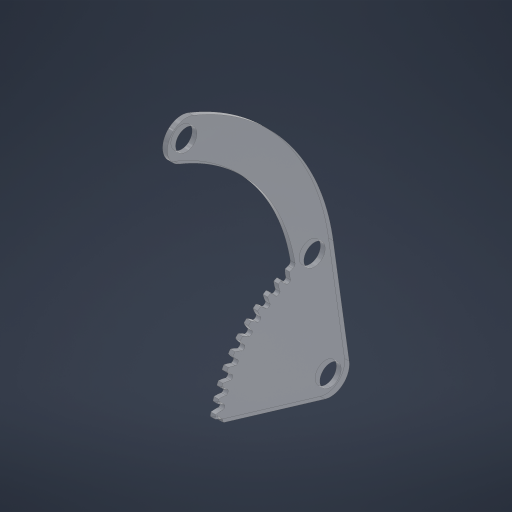
# Autodesk Inventor part: CORL_002_FanPlate
Saved by Autodesk Inventor 2024.2 (Build 282272000, 272)
## iProperties
Created: 2024-08-01
Part Number: CORL_002_FanPlate
Material: Polycarbonate, Clear
Document SubType Name: Modeling
Designer: Bryan
Mass: 349.383 g
Surface Area: 1019.32 cm^2
Volume: 291.153 cm^3
Density: 1.2 g/cm^3
Appearance: Polycarbonate - Clear
Author: Bryan
Autodesk Inventor part; units mm, degrees
ref_plane "YZ Plane" through (0, 0, 0) normal (1, 0, 0) x (0, 1, 0)
ref_plane "XZ Plane" through (0, 0, 0) normal (0, 1, 0) x (-1, 0, 0)
ref_plane "XY Plane" through (0, 0, 0) normal (0, 0, 1) x (1, 0, 0)
sketch "Sketch1" plane through (0, 0, 0) normal (1, 0, 0) x (0, 1, 0)
  circle A0 centre (0, 0) radius 152.4 construction
  circle A1 centre (0, 0) radius 157.48
  circle A2 centre (0, 0) radius 146.05
  line L0 (0, 0) -> (152.4, 0) construction
  line L1 (152.4, 0) -> (142.846, 36.9425) construction
  line L2 (142.846, 36.9425) -> (0, 0) construction
  arc A3 (147.5434, -0.8181) -> (142.846, 36.9425) centre (0, 0) ccw construction
  arc A4 (142.846, 36.9425) -> (137.6916, 53.0166) centre (0, 0) ccw construction
  line L3 (0, 0) -> (146, -3.8231) construction
  line L4 (137.6916, 53.0166) -> (157.4714, 1.6456) construction
  spline S0 degree 2 poles (157.4714, 1.6456) (152.4895, -0.3652) (147.5434, -0.8181) knots 0 0 0 1 1 1
  spline S1 degree 2 poles (157.1695, -9.8848) (152.2996, -7.616) (147.384, -6.9048) knots 0 0 0 1 1 1
  spline S2 degree 2 poles (156.4367, 18.0968) (151.6923, 15.5763) (146.8207, 14.6089) knots 0 0 0 1 1 1
  spline S3 degree 2 poles (157.3417, 6.5981) (152.2614, 8.3454) (147.2984, 8.5388) knots 0 0 0 1 1 1
  spline S4 degree 2 poles (153.6881, 34.3498) (149.2332, 31.3471) (144.4893, 29.8758) knots 0 0 0 1 1 1
  spline S5 degree 2 poles (155.7901, 23.0086) (150.555, 24.2153) (145.5989, 23.8889) knots 0 0 0 1 1 1
  spline S6 degree 2 poles (149.2557, 50.2264) (145.139, 46.7745) (140.575, 44.8154) knots 0 0 0 1 1 1
  spline S7 degree 2 poles (152.5316, 39.1671) (147.199, 39.8199) (142.3043, 38.9773) knots 0 0 0 1 1 1
  spline S8 degree 2 poles (143.188, 65.5527) (139.4546, 61.6895) (135.1204, 59.2639) knots 0 0 0 1 1 1
  spline S9 degree 2 poles (147.6019, 54.8964) (142.2303, 54.9883) (137.4505, 53.6386) knots 0 0 0 1 1 1
  spline S10 degree 2 poles (135.5514, 80.1608) (132.2424, 75.9285) (128.1854, 73.0632) knots 0 0 0 1 1 1
  spline S11 degree 2 poles (141.0551, 70.0243) (135.7033, 69.5542) (131.0907, 67.7123) knots 0 0 0 1 1 1
  spline S12 degree 2 poles (126.4298, 93.8907) (123.5812, 89.3356) (119.846, 86.062) knots 0 0 0 1 1 1
  spline S13 degree 2 poles (132.9629, 84.385) (127.6896, 83.358) (123.2948, 81.044) knots 0 0 0 1 1 1
  spline S14 degree 2 poles (115.9229, 106.5918) (113.5661, 101.764) (110.1936, 98.1178) knots 0 0 0 1 1 1
  spline S15 degree 2 poles (123.4139, 97.8211) (118.2768, 96.2485) (114.1479, 93.4879) knots 0 0 0 1 1 1
  spline S16 degree 2 poles (104.146, 118.1252) (102.3068, 113.0774) (99.3338, 109.0987) knots 0 0 0 1 1 1
  spline S17 degree 2 poles (112.5127, 110.1855) (107.5681, 108.0846) (103.7505, 104.9075) knots 0 0 0 1 1 1
  spline S18 degree 2 poles (91.2281, 128.3643) (89.9265, 123.1519) (87.3857, 118.8843) knots 0 0 0 1 1 1
  spline S19 degree 2 poles (100.3788, 121.3427) (95.6809, 118.7364) (92.2163, 115.1776) knots 0 0 0 1 1 1
  spline S20 degree 2 poles (77.3106, 137.197) (76.561, 131.8772) (74.4802, 127.3673) knots 0 0 0 1 1 1
  spline S21 degree 2 poles (87.1452, 131.1704) (82.7455, 128.0873) (79.6718, 124.1859) knots 0 0 0 1 1 1
  spline S22 degree 2 poles (62.5461, 144.5266) (62.3567, 139.1576) (60.7587, 134.4549) knots 0 0 0 1 1 1
  spline S23 degree 2 poles (72.9568, 139.561) (68.9034, 136.0349) (66.2544, 131.8336) knots 0 0 0 1 1 1
  spline S24 degree 2 poles (47.0963, 150.2727) (47.4691, 144.9133) (46.3715, 140.0693) knots 0 0 0 1 1 1
  spline S25 degree 2 poles (57.969, 146.4225) (54.3064, 142.4921) (52.1111, 138.0368) knots 0 0 0 1 1 1
  spline S26 degree 2 poles (31.1305, 154.3724) (32.0615, 149.0813) (31.4762, 144.1492) knots 0 0 0 1 1 1
  spline S27 degree 2 poles (42.3461, 151.6798) (39.1144, 147.3881) (37.3968, 142.7278) knots 0 0 0 1 1 1
  spline S28 degree 2 poles (14.8237, 156.7808) (16.3027, 151.616) (16.2361, 146.6497) knots 0 0 0 1 1 1
  spline S29 degree 2 poles (26.2593, 155.2752) (23.4939, 150.6692) (22.2728, 145.8549) knots 0 0 0 1 1 1
  spline S30 degree 2 poles (-1.6456, 157.4714) (0.3652, 152.4895) (0.8181, 147.5434) knots 0 0 0 1 1 1
  spline S31 degree 2 poles (9.8848, 157.1695) (7.616, 152.2996) (6.9048, 147.384) knots 0 0 0 1 1 1
  spline S32 degree 2 poles (-18.0968, 156.4367) (-15.5763, 151.6923) (-14.6089, 146.8207) knots 0 0 0 1 1 1
  spline S33 degree 2 poles (-6.5981, 157.3417) (-8.3454, 152.2614) (-8.5388, 147.2984) knots 0 0 0 1 1 1
  spline S34 degree 2 poles (-34.3498, 153.6881) (-31.3471, 149.2332) (-29.8758, 144.4893) knots 0 0 0 1 1 1
  spline S35 degree 2 poles (-23.0086, 155.7901) (-24.2153, 150.555) (-23.8889, 145.5989) knots 0 0 0 1 1 1
  spline S36 degree 2 poles (-50.2264, 149.2557) (-46.7745, 145.139) (-44.8154, 140.575) knots 0 0 0 1 1 1
  spline S37 degree 2 poles (-39.1671, 152.5316) (-39.8199, 147.199) (-38.9773, 142.3043) knots 0 0 0 1 1 1
  spline S38 degree 2 poles (-65.5527, 143.188) (-61.6895, 139.4546) (-59.2639, 135.1204) knots 0 0 0 1 1 1
  spline S39 degree 2 poles (-54.8964, 147.6019) (-54.9883, 142.2303) (-53.6386, 137.4505) knots 0 0 0 1 1 1
  spline S40 degree 2 poles (-80.1608, 135.5514) (-75.9285, 132.2424) (-73.0632, 128.1854) knots 0 0 0 1 1 1
  spline S41 degree 2 poles (-70.0243, 141.0551) (-69.5542, 135.7033) (-67.7123, 131.0907) knots 0 0 0 1 1 1
  spline S42 degree 2 poles (-93.8907, 126.4298) (-89.3356, 123.5812) (-86.062, 119.846) knots 0 0 0 1 1 1
  spline S43 degree 2 poles (-84.385, 132.9629) (-83.358, 127.6896) (-81.044, 123.2948) knots 0 0 0 1 1 1
  spline S44 degree 2 poles (-106.5918, 115.9229) (-101.764, 113.5661) (-98.1178, 110.1936) knots 0 0 0 1 1 1
  spline S45 degree 2 poles (-97.8211, 123.4139) (-96.2485, 118.2768) (-93.4879, 114.1479) knots 0 0 0 1 1 1
  spline S46 degree 2 poles (-118.1252, 104.146) (-113.0774, 102.3068) (-109.0987, 99.3338) knots 0 0 0 1 1 1
  spline S47 degree 2 poles (-110.1855, 112.5127) (-108.0846, 107.5681) (-104.9075, 103.7505) knots 0 0 0 1 1 1
  spline S48 degree 2 poles (-128.3643, 91.2281) (-123.1519, 89.9265) (-118.8843, 87.3857) knots 0 0 0 1 1 1
  spline S49 degree 2 poles (-121.3427, 100.3788) (-118.7364, 95.6809) (-115.1776, 92.2163) knots 0 0 0 1 1 1
  spline S50 degree 2 poles (-137.197, 77.3106) (-131.8772, 76.561) (-127.3673, 74.4802) knots 0 0 0 1 1 1
  spline S51 degree 2 poles (-131.1704, 87.1452) (-128.0873, 82.7455) (-124.1859, 79.6718) knots 0 0 0 1 1 1
  spline S52 degree 2 poles (-144.5266, 62.5461) (-139.1576, 62.3567) (-134.4549, 60.7587) knots 0 0 0 1 1 1
  spline S53 degree 2 poles (-139.561, 72.9568) (-136.0349, 68.9034) (-131.8336, 66.2544) knots 0 0 0 1 1 1
  spline S54 degree 2 poles (-150.2727, 47.0963) (-144.9133, 47.4691) (-140.0693, 46.3715) knots 0 0 0 1 1 1
  spline S55 degree 2 poles (-146.4225, 57.969) (-142.4921, 54.3064) (-138.0368, 52.1111) knots 0 0 0 1 1 1
  spline S56 degree 2 poles (-154.3724, 31.1305) (-149.0813, 32.0615) (-144.1492, 31.4762) knots 0 0 0 1 1 1
  spline S57 degree 2 poles (-151.6798, 42.3461) (-147.3881, 39.1144) (-142.7278, 37.3968) knots 0 0 0 1 1 1
  spline S58 degree 2 poles (-156.7808, 14.8237) (-151.616, 16.3027) (-146.6497, 16.2361) knots 0 0 0 1 1 1
  spline S59 degree 2 poles (-155.2752, 26.2593) (-150.6692, 23.4939) (-145.8549, 22.2728) knots 0 0 0 1 1 1
  spline S60 degree 2 poles (-157.4714, -1.6456) (-152.4895, 0.3652) (-147.5434, 0.8181) knots 0 0 0 1 1 1
  spline S61 degree 2 poles (-157.1695, 9.8848) (-152.2996, 7.616) (-147.384, 6.9048) knots 0 0 0 1 1 1
  spline S62 degree 2 poles (-156.4367, -18.0968) (-151.6923, -15.5763) (-146.8207, -14.6089) knots 0 0 0 1 1 1
  spline S63 degree 2 poles (-157.3417, -6.5981) (-152.2614, -8.3454) (-147.2984, -8.5388) knots 0 0 0 1 1 1
  spline S64 degree 2 poles (-153.6881, -34.3498) (-149.2332, -31.3471) (-144.4893, -29.8758) knots 0 0 0 1 1 1
  spline S65 degree 2 poles (-155.7901, -23.0086) (-150.555, -24.2153) (-145.5989, -23.8889) knots 0 0 0 1 1 1
  spline S66 degree 2 poles (-149.2557, -50.2264) (-145.139, -46.7745) (-140.575, -44.8154) knots 0 0 0 1 1 1
  spline S67 degree 2 poles (-152.5316, -39.1671) (-147.199, -39.8199) (-142.3043, -38.9773) knots 0 0 0 1 1 1
  spline S68 degree 2 poles (-143.188, -65.5527) (-139.4546, -61.6895) (-135.1204, -59.2639) knots 0 0 0 1 1 1
  spline S69 degree 2 poles (-147.6019, -54.8964) (-142.2303, -54.9883) (-137.4505, -53.6386) knots 0 0 0 1 1 1
  spline S70 degree 2 poles (-135.5514, -80.1608) (-132.2424, -75.9285) (-128.1854, -73.0632) knots 0 0 0 1 1 1
  spline S71 degree 2 poles (-141.0551, -70.0243) (-135.7033, -69.5542) (-131.0907, -67.7123) knots 0 0 0 1 1 1
  spline S72 degree 2 poles (-126.4298, -93.8907) (-123.5812, -89.3356) (-119.846, -86.062) knots 0 0 0 1 1 1
  spline S73 degree 2 poles (-132.9629, -84.385) (-127.6896, -83.358) (-123.2948, -81.044) knots 0 0 0 1 1 1
  spline S74 degree 2 poles (-115.9229, -106.5918) (-113.5661, -101.764) (-110.1936, -98.1178) knots 0 0 0 1 1 1
  spline S75 degree 2 poles (-123.4139, -97.8211) (-118.2768, -96.2485) (-114.1479, -93.4879) knots 0 0 0 1 1 1
  spline S76 degree 2 poles (-104.146, -118.1252) (-102.3068, -113.0774) (-99.3338, -109.0987) knots 0 0 0 1 1 1
  spline S77 degree 2 poles (-112.5127, -110.1855) (-107.5681, -108.0846) (-103.7505, -104.9075) knots 0 0 0 1 1 1
  spline S78 degree 2 poles (-91.2281, -128.3643) (-89.9265, -123.1519) (-87.3857, -118.8843) knots 0 0 0 1 1 1
  spline S79 degree 2 poles (-100.3788, -121.3427) (-95.6809, -118.7364) (-92.2163, -115.1776) knots 0 0 0 1 1 1
  spline S80 degree 2 poles (-77.3106, -137.197) (-76.561, -131.8772) (-74.4802, -127.3673) knots 0 0 0 1 1 1
  spline S81 degree 2 poles (-87.1452, -131.1704) (-82.7455, -128.0873) (-79.6718, -124.1859) knots 0 0 0 1 1 1
  spline S82 degree 2 poles (-62.5461, -144.5266) (-62.3567, -139.1576) (-60.7587, -134.4549) knots 0 0 0 1 1 1
  spline S83 degree 2 poles (-72.9568, -139.561) (-68.9034, -136.0349) (-66.2544, -131.8336) knots 0 0 0 1 1 1
  spline S84 degree 2 poles (-47.0963, -150.2727) (-47.4691, -144.9133) (-46.3715, -140.0693) knots 0 0 0 1 1 1
  spline S85 degree 2 poles (-57.969, -146.4225) (-54.3064, -142.4921) (-52.1111, -138.0368) knots 0 0 0 1 1 1
  spline S86 degree 2 poles (-31.1305, -154.3724) (-32.0615, -149.0813) (-31.4762, -144.1492) knots 0 0 0 1 1 1
  spline S87 degree 2 poles (-42.3461, -151.6798) (-39.1144, -147.3881) (-37.3968, -142.7278) knots 0 0 0 1 1 1
  spline S88 degree 2 poles (-14.8237, -156.7808) (-16.3027, -151.616) (-16.2361, -146.6497) knots 0 0 0 1 1 1
  spline S89 degree 2 poles (-26.2593, -155.2752) (-23.4939, -150.6692) (-22.2728, -145.8549) knots 0 0 0 1 1 1
  spline S90 degree 2 poles (1.6456, -157.4714) (-0.3652, -152.4895) (-0.8181, -147.5434) knots 0 0 0 1 1 1
  spline S91 degree 2 poles (-9.8848, -157.1695) (-7.616, -152.2996) (-6.9048, -147.384) knots 0 0 0 1 1 1
  spline S92 degree 2 poles (18.0968, -156.4367) (15.5763, -151.6923) (14.6089, -146.8207) knots 0 0 0 1 1 1
  spline S93 degree 2 poles (6.5981, -157.3417) (8.3454, -152.2614) (8.5388, -147.2984) knots 0 0 0 1 1 1
  spline S94 degree 2 poles (34.3498, -153.6881) (31.3471, -149.2332) (29.8758, -144.4893) knots 0 0 0 1 1 1
  spline S95 degree 2 poles (23.0086, -155.7901) (24.2153, -150.555) (23.8889, -145.5989) knots 0 0 0 1 1 1
  spline S96 degree 2 poles (50.2264, -149.2557) (46.7745, -145.139) (44.8154, -140.575) knots 0 0 0 1 1 1
  spline S97 degree 2 poles (39.1671, -152.5316) (39.8199, -147.199) (38.9773, -142.3043) knots 0 0 0 1 1 1
  spline S98 degree 2 poles (65.5527, -143.188) (61.6895, -139.4546) (59.2639, -135.1204) knots 0 0 0 1 1 1
  spline S99 degree 2 poles (54.8964, -147.6019) (54.9883, -142.2303) (53.6386, -137.4505) knots 0 0 0 1 1 1
  spline S100 degree 2 poles (80.1608, -135.5514) (75.9285, -132.2424) (73.0632, -128.1854) knots 0 0 0 1 1 1
  spline S101 degree 2 poles (70.0243, -141.0551) (69.5542, -135.7033) (67.7123, -131.0907) knots 0 0 0 1 1 1
  spline S102 degree 2 poles (93.8907, -126.4298) (89.3356, -123.5812) (86.062, -119.846) knots 0 0 0 1 1 1
  spline S103 degree 2 poles (84.385, -132.9629) (83.358, -127.6896) (81.044, -123.2948) knots 0 0 0 1 1 1
  spline S104 degree 2 poles (106.5918, -115.9229) (101.764, -113.5661) (98.1178, -110.1936) knots 0 0 0 1 1 1
  spline S105 degree 2 poles (97.8211, -123.4139) (96.2485, -118.2768) (93.4879, -114.1479) knots 0 0 0 1 1 1
  spline S106 degree 2 poles (118.1252, -104.146) (113.0774, -102.3068) (109.0987, -99.3338) knots 0 0 0 1 1 1
  spline S107 degree 2 poles (110.1855, -112.5127) (108.0846, -107.5681) (104.9075, -103.7505) knots 0 0 0 1 1 1
  spline S108 degree 2 poles (128.3643, -91.2281) (123.1519, -89.9265) (118.8843, -87.3857) knots 0 0 0 1 1 1
  spline S109 degree 2 poles (121.3427, -100.3788) (118.7364, -95.6809) (115.1776, -92.2163) knots 0 0 0 1 1 1
  spline S110 degree 2 poles (137.197, -77.3106) (131.8772, -76.561) (127.3673, -74.4802) knots 0 0 0 1 1 1
  spline S111 degree 2 poles (131.1704, -87.1452) (128.0873, -82.7455) (124.1859, -79.6718) knots 0 0 0 1 1 1
  spline S112 degree 2 poles (144.5266, -62.5461) (139.1576, -62.3567) (134.4549, -60.7587) knots 0 0 0 1 1 1
  spline S113 degree 2 poles (139.561, -72.9568) (136.0349, -68.9034) (131.8336, -66.2544) knots 0 0 0 1 1 1
  spline S114 degree 2 poles (150.2727, -47.0963) (144.9133, -47.4691) (140.0693, -46.3715) knots 0 0 0 1 1 1
  spline S115 degree 2 poles (146.4225, -57.969) (142.4921, -54.3064) (138.0368, -52.1111) knots 0 0 0 1 1 1
  spline S116 degree 2 poles (154.3724, -31.1305) (149.0813, -32.0615) (144.1492, -31.4762) knots 0 0 0 1 1 1
  spline S117 degree 2 poles (151.6798, -42.3461) (147.3881, -39.1144) (142.7278, -37.3968) knots 0 0 0 1 1 1
  spline S118 degree 2 poles (156.7808, -14.8237) (151.616, -16.3027) (146.6497, -16.2361) knots 0 0 0 1 1 1
  spline S119 degree 2 poles (155.2752, -26.2593) (150.6692, -23.4939) (145.8549, -22.2728) knots 0 0 0 1 1 1
  arc A5 (147.5434, -0.8181) -> (147.384, -6.9048) centre (149.8956, -3.9252) ccw
  arc A6 (146.8207, 14.6089) -> (147.2984, 8.5388) centre (149.4847, 11.7647) ccw
  arc A7 (144.4893, 29.8758) -> (145.5989, 23.8889) centre (147.4361, 27.3257) ccw
  arc A8 (140.575, 44.8154) -> (142.3043, 38.9773) centre (143.7721, 42.5872) ccw
  arc A9 (135.1204, 59.2639) -> (137.4505, 53.6386) centre (138.5329, 57.3822) ccw
  arc A10 (128.1854, 73.0632) -> (131.0907, 67.7123) centre (131.776, 71.5485) ccw
  arc A11 (119.846, 86.062) -> (123.2948, 81.044) centre (123.5752, 84.9309) ccw
  arc A12 (110.1936, 98.1178) -> (114.1479, 93.4879) centre (114.0206, 97.3828) ccw
  arc A13 (99.3338, 109.0987) -> (103.7505, 104.9075) centre (103.2167, 108.7677) ccw
  arc A14 (87.3857, 118.8843) -> (92.2163, 115.1776) centre (91.2819, 118.9609) ccw
  arc A15 (74.4802, 127.3673) -> (79.6718, 124.1859) centre (78.3471, 127.8508) ccw
  arc A16 (60.7587, 134.4549) -> (66.2544, 131.8336) centre (64.5538, 135.3399) ccw
  arc A17 (46.3715, 140.0693) -> (52.1111, 138.0368) centre (50.0533, 141.3462) ccw
  arc A18 (31.4762, 144.1492) -> (37.3968, 142.7278) centre (35.0044, 145.8039) ccw
  arc A19 (16.2361, 146.6497) -> (22.2728, 145.8549) centre (19.572, 148.6641) ccw
  arc A20 (0.8181, 147.5434) -> (6.9048, 147.384) centre (3.9252, 149.8956) ccw
  arc A21 (-14.6089, 146.8207) -> (-8.5388, 147.2984) centre (-11.7647, 149.4847) ccw
  arc A22 (-29.8758, 144.4893) -> (-23.8889, 145.5989) centre (-27.3257, 147.4361) ccw
  arc A23 (-44.8154, 140.575) -> (-38.9773, 142.3043) centre (-42.5872, 143.7721) ccw
  arc A24 (-59.2639, 135.1204) -> (-53.6386, 137.4505) centre (-57.3822, 138.5329) ccw
  arc A25 (-73.0632, 128.1854) -> (-67.7123, 131.0907) centre (-71.5485, 131.776) ccw
  arc A26 (-86.062, 119.846) -> (-81.044, 123.2948) centre (-84.9309, 123.5752) ccw
  arc A27 (-98.1178, 110.1936) -> (-93.4879, 114.1479) centre (-97.3828, 114.0206) ccw
  arc A28 (-109.0987, 99.3338) -> (-104.9075, 103.7505) centre (-108.7677, 103.2167) ccw
  arc A29 (-118.8843, 87.3857) -> (-115.1776, 92.2163) centre (-118.9609, 91.2819) ccw
  arc A30 (-127.3673, 74.4802) -> (-124.1859, 79.6718) centre (-127.8508, 78.3471) ccw
  arc A31 (-134.4549, 60.7587) -> (-131.8336, 66.2544) centre (-135.3399, 64.5538) ccw
  arc A32 (-140.0693, 46.3715) -> (-138.0368, 52.1111) centre (-141.3462, 50.0533) ccw
  arc A33 (-144.1492, 31.4762) -> (-142.7278, 37.3968) centre (-145.8039, 35.0044) ccw
  arc A34 (-146.6497, 16.2361) -> (-145.8549, 22.2728) centre (-148.6641, 19.572) ccw
  arc A35 (-147.5434, 0.8181) -> (-147.384, 6.9048) centre (-149.8956, 3.9252) ccw
  arc A36 (-146.8207, -14.6089) -> (-147.2984, -8.5388) centre (-149.4847, -11.7647) ccw
  arc A37 (-144.4893, -29.8758) -> (-145.5989, -23.8889) centre (-147.4361, -27.3257) ccw
  arc A38 (-140.575, -44.8154) -> (-142.3043, -38.9773) centre (-143.7721, -42.5872) ccw
  arc A39 (-135.1204, -59.2639) -> (-137.4505, -53.6386) centre (-138.5329, -57.3822) ccw
  arc A40 (-128.1854, -73.0632) -> (-131.0907, -67.7123) centre (-131.776, -71.5485) ccw
  arc A41 (-119.846, -86.062) -> (-123.2948, -81.044) centre (-123.5752, -84.9309) ccw
  arc A42 (-110.1936, -98.1178) -> (-114.1479, -93.4879) centre (-114.0206, -97.3828) ccw
  arc A43 (-99.3338, -109.0987) -> (-103.7505, -104.9075) centre (-103.2167, -108.7677) ccw
  arc A44 (-87.3857, -118.8843) -> (-92.2163, -115.1776) centre (-91.2819, -118.9609) ccw
  arc A45 (-74.4802, -127.3673) -> (-79.6718, -124.1859) centre (-78.3471, -127.8508) ccw
  arc A46 (-60.7587, -134.4549) -> (-66.2544, -131.8336) centre (-64.5538, -135.3399) ccw
  arc A47 (-46.3715, -140.0693) -> (-52.1111, -138.0368) centre (-50.0533, -141.3462) ccw
  arc A48 (-31.4762, -144.1492) -> (-37.3968, -142.7278) centre (-35.0044, -145.8039) ccw
  arc A49 (-16.2361, -146.6497) -> (-22.2728, -145.8549) centre (-19.572, -148.6641) ccw
  arc A50 (-0.8181, -147.5434) -> (-6.9048, -147.384) centre (-3.9252, -149.8956) ccw
  arc A51 (14.6089, -146.8207) -> (8.5388, -147.2984) centre (11.7647, -149.4847) ccw
  arc A52 (29.8758, -144.4893) -> (23.8889, -145.5989) centre (27.3257, -147.4361) ccw
  arc A53 (44.8154, -140.575) -> (38.9773, -142.3043) centre (42.5872, -143.7721) ccw
  arc A54 (59.2639, -135.1204) -> (53.6386, -137.4505) centre (57.3822, -138.5329) ccw
  arc A55 (73.0632, -128.1854) -> (67.7123, -131.0907) centre (71.5485, -131.776) ccw
  arc A56 (86.062, -119.846) -> (81.044, -123.2948) centre (84.9309, -123.5752) ccw
  arc A57 (98.1178, -110.1936) -> (93.4879, -114.1479) centre (97.3828, -114.0206) ccw
  arc A58 (109.0987, -99.3338) -> (104.9075, -103.7505) centre (108.7677, -103.2167) ccw
  arc A59 (118.8843, -87.3857) -> (115.1776, -92.2163) centre (118.9609, -91.2819) ccw
  arc A60 (127.3673, -74.4802) -> (124.1859, -79.6718) centre (127.8508, -78.3471) ccw
  arc A61 (134.4549, -60.7587) -> (131.8336, -66.2544) centre (135.3399, -64.5538) ccw
  arc A62 (140.0693, -46.3715) -> (138.0368, -52.1111) centre (141.3462, -50.0533) ccw
  arc A63 (144.1492, -31.4762) -> (142.7278, -37.3968) centre (145.8039, -35.0044) ccw
  arc A64 (146.6497, -16.2361) -> (145.8549, -22.2728) centre (148.6641, -19.572) ccw
  point P0 (152.1911, -7.976)
  point P1 (151.5651, 15.9301)
  point P2 (152.1911, 7.976)
  point P3 (149.0697, 31.6857)
  point P4 (150.5237, 23.8406)
  point P5 (144.941, 47.0942)
  point P6 (147.2071, 39.444)
  point P7 (139.2243, 61.9867)
  point P8 (142.2777, 54.6153)
  point P9 (131.9823, 76.2)
  point P10 (135.7894, 69.1882)
  point P11 (123.2942, 89.5785)
  point P12 (127.8134, 83.003)
  point P13 (113.2553, 101.9755)
  point P14 (118.437, 95.9084)
  point P15 (101.9755, 113.2553)
  point P16 (107.7631, 107.7631)
  point P17 (89.5785, 123.2942)
  point P18 (95.9084, 118.437)
  point P19 (76.2, 131.9823)
  point P20 (83.003, 127.8134)
  point P21 (61.9867, 139.2243)
  point P22 (69.1882, 135.7894)
  point P23 (47.0942, 144.941)
  point P24 (54.6153, 142.2777)
  point P25 (31.6857, 149.0697)
  point P26 (39.444, 147.2071)
  point P27 (15.9301, 151.5651)
  point P28 (23.8406, 150.5237)
  point P29 (0, 152.4)
  point P30 (7.976, 152.1911)
  point P31 (-15.9301, 151.5651)
  point P32 (-7.976, 152.1911)
  point P33 (-31.6857, 149.0697)
  point P34 (-23.8406, 150.5237)
  point P35 (-47.0942, 144.941)
  point P36 (-39.444, 147.2071)
  point P37 (-61.9867, 139.2243)
  point P38 (-54.6153, 142.2777)
  point P39 (-76.2, 131.9823)
  point P40 (-69.1882, 135.7894)
  point P41 (-89.5785, 123.2942)
  point P42 (-83.003, 127.8134)
  point P43 (-101.9755, 113.2553)
  point P44 (-95.9084, 118.437)
  point P45 (-113.2553, 101.9755)
  point P46 (-107.7631, 107.7631)
  point P47 (-123.2942, 89.5785)
  point P48 (-118.437, 95.9084)
  point P49 (-131.9823, 76.2)
  point P50 (-127.8134, 83.003)
  point P51 (-139.2243, 61.9867)
  point P52 (-135.7894, 69.1882)
  point P53 (-144.941, 47.0942)
  point P54 (-142.2777, 54.6153)
  point P55 (-149.0697, 31.6857)
  point P56 (-147.2071, 39.444)
  point P57 (-151.5651, 15.9301)
  point P58 (-150.5237, 23.8406)
  point P59 (-152.4, 0)
  point P60 (-152.1911, 7.976)
  point P61 (-151.5651, -15.9301)
  point P62 (-152.1911, -7.976)
  point P63 (-149.0697, -31.6857)
  point P64 (-150.5237, -23.8406)
  point P65 (-144.941, -47.0942)
  point P66 (-147.2071, -39.444)
  point P67 (-139.2243, -61.9867)
  point P68 (-142.2777, -54.6153)
  point P69 (-131.9823, -76.2)
  point P70 (-135.7894, -69.1882)
  point P71 (-123.2942, -89.5785)
  point P72 (-127.8134, -83.003)
  point P73 (-113.2553, -101.9755)
  point P74 (-118.437, -95.9084)
  point P75 (-101.9755, -113.2553)
  point P76 (-107.7631, -107.7631)
  point P77 (-89.5785, -123.2942)
  point P78 (-95.9084, -118.437)
  point P79 (-76.2, -131.9823)
  point P80 (-83.003, -127.8134)
  point P81 (-61.9867, -139.2243)
  point P82 (-69.1882, -135.7894)
  point P83 (-47.0942, -144.941)
  point P84 (-54.6153, -142.2777)
  point P85 (-31.6857, -149.0697)
  point P86 (-39.444, -147.2071)
  point P87 (-15.9301, -151.5651)
  point P88 (-23.8406, -150.5237)
  point P89 (0, -152.4)
  point P90 (-7.976, -152.1911)
  point P91 (15.9301, -151.5651)
  point P92 (7.976, -152.1911)
  point P93 (31.6857, -149.0697)
  point P94 (23.8406, -150.5237)
  point P95 (47.0942, -144.941)
  point P96 (39.444, -147.2071)
  point P97 (61.9867, -139.2243)
  point P98 (54.6153, -142.2777)
  point P99 (76.2, -131.9823)
  point P100 (69.1882, -135.7894)
  point P101 (89.5785, -123.2942)
  point P102 (83.003, -127.8134)
  point P103 (101.9755, -113.2553)
  point P104 (95.9084, -118.437)
  point P105 (113.2553, -101.9755)
  point P106 (107.7631, -107.7631)
  point P107 (123.2942, -89.5785)
  point P108 (118.437, -95.9084)
  point P109 (131.9823, -76.2)
  point P110 (127.8134, -83.003)
  point P111 (139.2243, -61.9867)
  point P112 (135.7894, -69.1882)
  point P113 (144.941, -47.0942)
  point P114 (142.2777, -54.6153)
  point P115 (149.0697, -31.6857)
  point P116 (147.2071, -39.444)
  point P117 (151.5651, -15.9301)
  point P118 (150.5237, -23.8406)
  point P119 (-110.1573, 193.0296)
  point P120 (-157.4714, -1.6456)
  point P121 (157.1695, -9.8848)
  point P122 (222.1508, -6.6412)
  point P123 (222.2472, -1.1158)
  point P124 (157.3417, 6.5981)
  point P125 (222.0729, 8.8715)
  point P126 (221.7837, 14.3901)
  point P127 (155.7901, 23.0086)
  point P128 (220.9131, 24.3409)
  point P129 (220.2396, 29.8259)
  point P130 (152.5316, 39.1671)
  point P131 (218.677, 39.6917)
  point P132 (217.6226, 45.1163)
  point P133 (149.2557, 50.2264)
  point P134 (147.6019, 54.8964)
  point P135 (215.3756, 54.8491)
  point P136 (213.9453, 60.187)
  point P137 (143.188, 65.5527)
  point P138 (141.0551, 70.0243)
  point P139 (211.0248, 69.7394)
  point P140 (209.2257, 74.9645)
  point P141 (135.5514, 80.1608)
  point P142 (132.9629, 84.385)
  point P143 (205.646, 84.2898)
  point P144 (203.4868, 89.3767)
  point P145 (126.4298, 93.8907)
  point P146 (123.4139, 97.8211)
  point P147 (199.2653, 98.4297)
  point P148 (196.7565, 103.3535)
  point P149 (115.9229, 106.5918)
  point P150 (112.5127, 110.1855)
  point P151 (191.9138, 112.0899)
  point P152 (189.0676, 116.8268)
  point P153 (104.146, 118.1252)
  point P154 (100.3788, 121.3427)
  point P155 (183.6273, 125.2041)
  point P156 (180.4576, 129.7309)
  point P157 (91.2281, 128.3643)
  point P158 (87.1452, 131.1704)
  point P159 (174.4462, 137.7083)
  point P160 (170.9685, 142.003)
  point P161 (77.3106, 137.197)
  point P162 (72.9568, 139.561)
  point P163 (164.4152, 149.5416)
  point P164 (160.6464, 153.5832)
  point P165 (62.5461, 144.5266)
  point P166 (57.969, 146.4225)
  point P167 (153.5832, 160.6464)
  point P168 (149.5416, 164.4152)
  point P169 (47.0963, 150.2727)
  point P170 (42.3461, 151.6798)
  point P171 (142.003, 170.9685)
  point P172 (137.7083, 174.4462)
  point P173 (31.1305, 154.3724)
  point P174 (26.2593, 155.2752)
  point P175 (129.7309, 180.4576)
  point P176 (125.2041, 183.6273)
  point P177 (14.8237, 156.7808)
  point P178 (9.8848, 157.1695)
  point P179 (116.8268, 189.0676)
  point P180 (112.0899, 191.9138)
  point P181 (-1.6456, 157.4714)
  point P182 (-6.5981, 157.3417)
  point P183 (103.3535, 196.7565)
  point P184 (98.4297, 199.2653)
  point P185 (-18.0968, 156.4367)
  point P186 (-23.0086, 155.7901)
  point P187 (89.3767, 203.4868)
  point P188 (84.2898, 205.646)
  point P189 (-34.3498, 153.6881)
  point P190 (-39.1671, 152.5316)
  point P191 (74.9645, 209.2257)
  point P192 (69.7394, 211.0248)
  point P193 (-54.8964, 147.6019)
  point P194 (60.187, 213.9453)
  point P195 (54.8491, 215.3756)
  point P196 (-65.5527, 143.188)
  point P197 (-70.0243, 141.0551)
  point P198 (45.1163, 217.6226)
  point P199 (39.6917, 218.677)
  dimension "d18" = 304.8
  dimension "d19" = 314.96
  dimension "d20" = 292.1
  dimension "d21" = 14.5
  dimension "d22" = 38.1579
  dimension "d23" = 38.1579
  dimension "d26" = 1.5
  dimension "d61" = 55.0474
  dimension "d62" = 16.8895
  dimension "d65" = 360
  dimension "d104" = 360
  constraints: 184 point on circle, 62 centre point, 10 end point, 3 coincident, 3 symmetric about line, 2 tangent, 1 horizontal, 1 horizontal alignment, 1 perpendicular, 1154 other
  measures "d21" angle of L0 L2
  measures "d22" distance of L0.end L1.end
  measures "d26" angle of L3 L0
  measures "d61" distance of L4.start L4.end
extrude "Extrusion2" add sketch "Sketch1" along normal blind 6.35 contours S0 A5 A2 A6 S3 A1 | A1 S118 A64 A2 A5 S1 | S2 A6 A2 A7 S5 A1 | A2 | A1 S116 A63 A2 A64 S119 | S4 A7 A2 A8 S7 A1 | A63 S117 A1 S114 A62 A2 | A2 A9 S9 A1 S6 A8 | A62 S115 A1 S112 A61 A2 | A2 A10 S11 A1 S8 A9 | A61 S113 A1 S110 A60 A2 | A2 A11 S13 A1 S10 A10 | A60 S111 A1 S108 A59 A2 | A60 S110 A1 S111 | A2 A12 S15 A1 S12 A11 | A59 S109 A1 S106 A58 A2 | A59 S108 A1 S109 | A2 A13 S17 A1 S14 A12 | A58 S107 A1 S104 A57 A2 | A58 S106 A1 S107 | A2 A14 S19 A1 S16 A13 | A57 S105 A1 S102 A56 A2 | A57 S104 A1 S105 | A2 A15 S21 A1 S18 A14 | A56 S103 A1 S100 A55 A2 | A56 S102 A1 S103 | A2 A16 S23 A1 S20 A15 | A55 S101 A1 S98 A54 A2 | A55 S100 A1 S101 | A2 A17 S25 A1 S22 A16 | A54 S99 A1 S96 A53 A2 | A54 S98 A1 S99 | A2 A18 S27 A1 S24 A17 | A53 S97 A1 S94 A52 A2 | A53 S96 A1 S97 | A2 A19 S29 A1 S26 A18 | A52 S95 A1 S92 A51 A2 | A52 S94 A1 S95 | A2 A20 S31 A1 S28 A19 | A51 S93 A1 S90 A50 A2 | A51 S92 A1 S93 | A2 A21 S33 A1 S30 A20 | A50 S91 A1 S88 A49 A2 | A50 S90 A1 S91 | A2 A22 S35 A1 S32 A21 | A49 S89 A1 S86 A48 A2 | A49 S88 A1 S89 | A2 A23 S37 A1 S34 A22 | A22 S34 A1 S35 | A48 S87 A1 S84 A47 A2 | A48 S86 A1 S87 | A2 A24 S39 A1 S36 A23 | A23 S36 A1 S37 | A47 S85 A1 S82 A46 A2 | A47 S84 A1 S85 | A2 A25 S41 A1 S38 A24 | A24 S38 A1 S39 | A46 S83 A1 S80 A45 A2 | A46 S82 A1 S83 | A2 A26 S43 A1 S40 A25 | A25 S40 A1 S41 | A45 S81 A1 S78 A44 A2 | A45 S80 A1 S81 | A2 A27 S45 A1 S42 A26 | A26 S42 A1 S43 | A44 S79 A1 S76 A43 A2 | A44 S78 A1 S79 | A2 A28 S47 A1 S44 A27 | A27 S44 A1 S45 | A43 S77 A1 S74 A42 A2 | A43 S76 A1 S77 | A2 A29 S49 A1 S46 A28 | A28 S46 A1 S47 | A42 S75 A1 S72 A41 A2 | A42 S74 A1 S75 | A2 A30 S51 A1 S48 A29 | A29 S48 A1 S49 | A41 S73 A1 S70 A40 A2 | A41 S72 A1 S73 | A2 A31 S53 A1 S50 A30 | A30 S50 A1 S51 | A40 S71 A1 S68 A39 A2 | A40 S70 A1 S71 | A2 A32 S55 A1 S52 A31 | A31 S52 A1 S53 | A39 S69 A1 S66 A38 A2 | A39 S68 A1 S69 | A2 A33 S57 A1 S54 A32 | A32 S54 A1 S55 | A38 S67 A1 S64 A37 A2 | A38 S66 A1 S67 | A2 A34 S59 A1 S56 A33 | A33 S56 A1 S57 | A37 S65 A1 S62 A36 A2 | A37 S64 A1 S65 | A2 A35 S61 A1 S58 A34 | A34 S58 A1 S59 | A36 S63 A1 S60 A35 A2 | A36 S62 A1 S63 | A35 S60 A1 S61
sketch "Sketch11" plane through (6.35, 0, 0) normal (1, 0, 0) x (0, 0, -1)
  arc A0 (-1.6456, 157.4714) -> (-6.5981, 157.3417) centre (0, 0) ccw projected
  arc A1 (0.8181, 147.5434) -> (6.9048, 147.384) centre (3.9252, 149.8956) ccw projected
  line L0 (3.8231, 146) -> (0, 0) construction
  line L1 (0, 0) -> (-156.4677, 17.8272) construction
  circle A2 centre (0, 0) radius 157.48
  arc A3 (-146.6497, 16.2361) -> (-145.8549, 22.2728) centre (-148.6641, 19.572) ccw projected
  arc A4 (-156.4367, -18.0968) -> (72.9568, 139.561) centre (0, 0) ccw projected
  arc A5 (60.7587, 134.4549) -> (66.2544, 131.8336) centre (64.5538, 135.3399) ccw projected
  arc A6 (62.5461, 144.5266) -> (57.969, 146.4225) centre (0, 0) ccw projected
  arc A7 (46.3715, 140.0693) -> (52.1111, 138.0368) centre (50.0533, 141.3462) ccw projected
  arc A8 (47.0963, 150.2727) -> (42.3461, 151.6798) centre (0, 0) ccw projected
  arc A9 (31.4762, 144.1492) -> (37.3968, 142.7278) centre (35.0044, 145.8039) ccw projected
  arc A10 (31.1305, 154.3724) -> (26.2593, 155.2752) centre (0, 0) ccw projected
  arc A11 (16.2361, 146.6497) -> (22.2728, 145.8549) centre (19.572, 148.6641) ccw projected
  arc A12 (14.8237, 156.7808) -> (9.8848, 157.1695) centre (0, 0) ccw projected
  arc A13 (0.8181, 147.5434) -> (6.9048, 147.384) centre (3.9252, 149.8956) ccw projected
  spline S0 degree 2 poles (0.8181, 147.5434) (0.3652, 152.4895) (-1.6456, 157.4714) knots 0 0 0 1 1 1 projected
  arc A14 (-1.6456, 157.4714) -> (-6.5981, 157.3417) centre (0, 0) ccw projected
  spline S1 degree 2 poles (-6.5981, 157.3417) (-8.3454, 152.2614) (-8.5388, 147.2984) knots 0 0 0 1 1 1 projected
  arc A15 (-14.6089, 146.8207) -> (-8.5388, 147.2984) centre (-11.7647, 149.4847) ccw projected
  spline S2 degree 2 poles (-14.6089, 146.8207) (-15.5763, 151.6923) (-18.0968, 156.4367) knots 0 0 0 1 1 1 projected
  arc A16 (-18.0968, 156.4367) -> (-23.0086, 155.7901) centre (0, 0) ccw projected
  spline S3 degree 2 poles (-23.0086, 155.7901) (-24.2153, 150.555) (-23.8889, 145.5989) knots 0 0 0 1 1 1 projected
  arc A17 (-29.8758, 144.4893) -> (-23.8889, 145.5989) centre (-27.3257, 147.4361) ccw projected
  spline S4 degree 2 poles (-29.8758, 144.4893) (-31.3471, 149.2332) (-34.3498, 153.6881) knots 0 0 0 1 1 1 projected
  arc A18 (-34.3498, 153.6881) -> (-39.1671, 152.5316) centre (0, 0) ccw projected
  spline S5 degree 2 poles (-39.1671, 152.5316) (-39.8199, 147.199) (-38.9773, 142.3043) knots 0 0 0 1 1 1 projected
  arc A19 (-44.8154, 140.575) -> (-38.9773, 142.3043) centre (-42.5872, 143.7721) ccw projected
  spline S6 degree 2 poles (-44.8154, 140.575) (-46.7745, 145.139) (-50.2264, 149.2557) knots 0 0 0 1 1 1 projected
  arc A20 (-50.2264, 149.2557) -> (-54.8964, 147.6019) centre (0, 0) ccw projected
  spline S7 degree 2 poles (-54.8964, 147.6019) (-54.9883, 142.2303) (-53.6386, 137.4505) knots 0 0 0 1 1 1 projected
  arc A21 (-59.2639, 135.1204) -> (-53.6386, 137.4505) centre (-57.3822, 138.5329) ccw projected
  spline S8 degree 2 poles (-59.2639, 135.1204) (-61.6895, 139.4546) (-65.5527, 143.188) knots 0 0 0 1 1 1 projected
  arc A22 (-65.5527, 143.188) -> (-70.0243, 141.0551) centre (0, 0) ccw projected
  spline S9 degree 2 poles (-70.0243, 141.0551) (-69.5542, 135.7033) (-67.7123, 131.0907) knots 0 0 0 1 1 1 projected
  arc A23 (-73.0632, 128.1854) -> (-67.7123, 131.0907) centre (-71.5485, 131.776) ccw projected
  spline S10 degree 2 poles (-73.0632, 128.1854) (-75.9285, 132.2424) (-80.1608, 135.5514) knots 0 0 0 1 1 1 projected
  arc A24 (-80.1608, 135.5514) -> (-84.385, 132.9629) centre (0, 0) ccw projected
  spline S11 degree 2 poles (-84.385, 132.9629) (-83.358, 127.6896) (-81.044, 123.2948) knots 0 0 0 1 1 1 projected
  arc A25 (-86.062, 119.846) -> (-81.044, 123.2948) centre (-84.9309, 123.5752) ccw projected
  spline S12 degree 2 poles (-86.062, 119.846) (-89.3356, 123.5812) (-93.8907, 126.4298) knots 0 0 0 1 1 1 projected
  arc A26 (-93.8907, 126.4298) -> (-97.8211, 123.4139) centre (0, 0) ccw projected
  spline S13 degree 2 poles (-97.8211, 123.4139) (-96.2485, 118.2768) (-93.4879, 114.1479) knots 0 0 0 1 1 1 projected
  arc A27 (-98.1178, 110.1936) -> (-93.4879, 114.1479) centre (-97.3828, 114.0206) ccw projected
  spline S14 degree 2 poles (-98.1178, 110.1936) (-101.764, 113.5661) (-106.5918, 115.9229) knots 0 0 0 1 1 1 projected
  arc A28 (-106.5918, 115.9229) -> (-110.1855, 112.5127) centre (0, 0) ccw projected
  spline S15 degree 2 poles (-110.1855, 112.5127) (-108.0846, 107.5681) (-104.9075, 103.7505) knots 0 0 0 1 1 1 projected
  arc A29 (-109.0987, 99.3338) -> (-104.9075, 103.7505) centre (-108.7677, 103.2167) ccw projected
  spline S16 degree 2 poles (-109.0987, 99.3338) (-113.0774, 102.3068) (-118.1252, 104.146) knots 0 0 0 1 1 1 projected
  arc A30 (-118.1252, 104.146) -> (-121.3427, 100.3788) centre (0, 0) ccw projected
  spline S17 degree 2 poles (-121.3427, 100.3788) (-118.7364, 95.6809) (-115.1776, 92.2163) knots 0 0 0 1 1 1 projected
  arc A31 (-118.8843, 87.3857) -> (-115.1776, 92.2163) centre (-118.9609, 91.2819) ccw projected
  spline S18 degree 2 poles (-118.8843, 87.3857) (-123.1519, 89.9265) (-128.3643, 91.2281) knots 0 0 0 1 1 1 projected
  arc A32 (-128.3643, 91.2281) -> (-131.1704, 87.1452) centre (0, 0) ccw projected
  spline S19 degree 2 poles (-131.1704, 87.1452) (-128.0873, 82.7455) (-124.1859, 79.6718) knots 0 0 0 1 1 1 projected
  arc A33 (-127.3673, 74.4802) -> (-124.1859, 79.6718) centre (-127.8508, 78.3471) ccw projected
  spline S20 degree 2 poles (-127.3673, 74.4802) (-131.8772, 76.561) (-137.197, 77.3106) knots 0 0 0 1 1 1 projected
  arc A34 (-137.197, 77.3106) -> (-139.561, 72.9568) centre (0, 0) ccw projected
  spline S21 degree 2 poles (-139.561, 72.9568) (-136.0349, 68.9034) (-131.8336, 66.2544) knots 0 0 0 1 1 1 projected
  arc A35 (-134.4549, 60.7587) -> (-131.8336, 66.2544) centre (-135.3399, 64.5538) ccw projected
  spline S22 degree 2 poles (-134.4549, 60.7587) (-139.1576, 62.3567) (-144.5266, 62.5461) knots 0 0 0 1 1 1 projected
  arc A36 (-144.5266, 62.5461) -> (-146.4225, 57.969) centre (0, 0) ccw projected
  spline S23 degree 2 poles (-146.4225, 57.969) (-142.4921, 54.3064) (-138.0368, 52.1111) knots 0 0 0 1 1 1 projected
  arc A37 (-140.0693, 46.3715) -> (-138.0368, 52.1111) centre (-141.3462, 50.0533) ccw projected
  spline S24 degree 2 poles (-140.0693, 46.3715) (-144.9133, 47.4691) (-150.2727, 47.0963) knots 0 0 0 1 1 1 projected
  arc A38 (-150.2727, 47.0963) -> (-151.6798, 42.3461) centre (0, 0) ccw projected
  spline S25 degree 2 poles (-151.6798, 42.3461) (-147.3881, 39.1144) (-142.7278, 37.3968) knots 0 0 0 1 1 1 projected
  arc A39 (-144.1492, 31.4762) -> (-142.7278, 37.3968) centre (-145.8039, 35.0044) ccw projected
  spline S26 degree 2 poles (-144.1492, 31.4762) (-149.0813, 32.0615) (-154.3724, 31.1305) knots 0 0 0 1 1 1 projected
  arc A40 (-154.3724, 31.1305) -> (-155.2752, 26.2593) centre (0, 0) ccw projected
  spline S27 degree 2 poles (-155.2752, 26.2593) (-150.6692, 23.4939) (-145.8549, 22.2728) knots 0 0 0 1 1 1 projected
  arc A41 (-146.6497, 16.2361) -> (-145.8549, 22.2728) centre (-148.6641, 19.572) ccw projected
  arc A42 (-156.7808, 14.8237) -> (-157.1695, 9.8848) centre (0, 0) ccw projected
  arc A43 (-147.5434, 0.8181) -> (-147.384, 6.9048) centre (-149.8956, 3.9252) ccw projected
  arc A44 (-157.4714, -1.6456) -> (-157.3417, -6.5981) centre (0, 0) ccw projected
  arc A45 (-146.8207, -14.6089) -> (-147.2984, -8.5388) centre (-149.4847, -11.7647) ccw projected
  arc A46 (-144.1492, 31.4762) -> (-142.7278, 37.3968) centre (-145.8039, 35.0044) ccw projected
  circle A47 centre (0, 0) radius 14.2875
  circle A48 centre (0, 0) radius 25.4
  line L2 (-143.0357, 16.3365) -> (-7.2895, -24.3315)
  line L3 (3.8231, 146) -> (25.12, 3.7611)
  line L4 (-144.8005, 19.0634) -> (-145.1333, 16.5358) construction
  arc A49 (-144.8005, 19.0634) -> (-142.6003, 16.2473) centre (-142.3168, 18.7364) ccw
  point P0 (57.969, 146.4225)
  point P1 (47.0963, 150.2727)
  point P2 (42.3461, 151.6798)
  point P3 (31.1305, 154.3724)
  point P4 (26.2593, 155.2752)
  point P5 (14.8237, 156.7808)
  point P6 (9.8848, 157.1695)
  point P7 (6.9048, 147.384)
  point P8 (-146.6497, 16.2361)
  point P9 (-156.7808, 14.8237)
  point P10 (-157.1695, 9.8848)
  point P11 (-157.4714, -1.6456)
  point P12 (-157.3417, -6.5981)
  point P13 (72.9568, 139.561)
  point P14 (-146.0914, 16.645)
  point P15 (-151.6798, 42.3461)
  point P16 (-146.4225, 57.969)
  point P17 (-139.561, 72.9568)
  point P18 (-131.1704, 87.1452)
  point P19 (-121.3427, 100.3788)
  point P20 (-110.1855, 112.5127)
  point P21 (-97.8211, 123.4139)
  point P22 (-84.385, 132.9629)
  point P23 (-70.0243, 141.0551)
  point P24 (-54.8964, 147.6019)
  point P25 (-39.1671, 152.5316)
  point P26 (-50.2264, 149.2557)
  point P27 (-23.0086, 155.7901)
  point P28 (-34.3498, 153.6881)
  point P29 (-1.6456, 157.4714)
  point P30 (-155.2752, 26.2593)
  point P31 (-6.5981, 157.3417)
  point P32 (-18.0968, 156.4367)
  point P33 (26.2593, 155.2752)
  point P34 (14.8237, 156.7808)
  point P35 (9.8848, 157.1695)
  point P36 (-156.7808, 14.8237)
  point P37 (-157.1695, 9.8848)
  point P38 (-157.4714, -1.6456)
  point P39 (-157.3417, -6.5981)
  point P40 (72.9568, 139.561)
  point P41 (57.969, 146.4225)
  point P42 (47.0963, 150.2727)
  point P43 (42.3461, 151.6798)
  point P44 (31.1305, 154.3724)
  point P45 (-153.6233, 31.255)
  point P46 (0.8181, 147.5434)
  point P47 (0.6649, 25.3913)
  point P48 (-25.2367, 2.8754)
  point P49 (-151.6798, 42.3461)
  point P50 (-155.2752, 26.2593)
  point P51 (-1.6456, 157.4714)
  point P52 (-6.5981, 157.3417)
  point P53 (-18.0968, 156.4367)
  point P54 (-23.0086, 155.7901)
  point P55 (-34.3498, 153.6881)
  point P56 (-39.1671, 152.5316)
  point P57 (-50.2264, 149.2557)
  point P58 (-54.8964, 147.6019)
  point P59 (-70.0243, 141.0551)
  point P60 (-84.385, 132.9629)
  point P61 (-97.8211, 123.4139)
  point P62 (-110.1855, 112.5127)
  point P63 (-121.3427, 100.3788)
  point P64 (-131.1704, 87.1452)
  point P65 (-139.561, 72.9568)
  point P66 (-146.4225, 57.969)
  point P67 (-145.8549, 22.2728)
  dimension "d106" = 314.96
  dimension "d107" = 85
  dimension "d108" = 28.575
  dimension "d109" = 50.8
  constraints: 10 end point, 9 point on circle, 6 tangent, 3 centre point, 3 coincident, 3 point on line, 44 other
  measures "d107" angle of L0 L1
  measures "d108" diameter of A47
  measures "d109" diameter of A48
extrude "Extrusion12" cut sketch "Sketch11" against normal blind 6.35 contours A2 S27 A3 A49 L2 A48 L3 A1 S0 | S1 A15 S2 A2 | S3 A17 S4 A2 | S5 A19 S6 A2 | S7 A21 S8 A2 | S9 A23 S10 A2 | A2 S25 A39 S26 | S11 A25 S12 A2 | A2 S23 A37 S24 | S13 A27 S14 A2 | A2 S21 A35 S22 | S15 A29 S16 A2 | A2 S19 A33 S20 | S17 A31 S18 A2 | A47
sketch "Sketch14" plane through (6.35, 0, 0) normal (1, 0, 0) x (0, 0, -1)
  arc A0 (0.8181, 147.5434) -> (3.8231, 146) centre (3.9252, 149.8956) ccw projected
  line L0 (0, 0) -> (3.8231, 146) construction
  line L1 (0, 0) -> (-47.8481, 150.035) construction
  arc A1 (-50.2264, 149.2557) -> (-54.8964, 147.6019) centre (0, 0) ccw projected
  circle A2 centre (-21.4577, 150.8818) radius 25.4
  circle A3 centre (-21.4577, 150.8818) radius 14.2875
  dimension "d110" = 19.188
  dimension "d111" = 50.8
  dimension "d112" = 28.575
  constraints: 4 end point, 2 centre point, 2 tangent, 1 coincident, 1 point on circle
  measures "d110" angle of L0 L1
  measures "d111" diameter of A2
  measures "d112" diameter of A3
extrude "Extrusion14" add sketch "Sketch14" against normal blind 6.35
extrude "Extrusion15" cut sketch "Sketch14" against normal blind 6.35 contours A3
sketch "Sketch17" plane through (6.35, 0, 0) normal (1, 0, 0) x (0, 0, -1)
  arc A0 (3.4736, 146.0249) -> (-44.6138, 140.4435) centre (-21.4577, 150.8818) ccw projected
  arc A1 (-50.2264, 149.2557) -> (-46.7086, 153.6299) centre (-51.8881, 154.1936) ccw
  arc A2 (-50.2264, 149.2557) -> (-54.8964, 147.6019) centre (0, 0) ccw projected
  circle A3 centre (-21.4577, 150.8818) radius 14.2875 projected
  circle A4 centre (0, 0) radius 14.2875 projected
  arc A5 (3.4736, 146.0249) -> (-44.6138, 140.4435) centre (-21.4577, 150.8818) ccw projected
  arc A6 (-44.8154, 140.575) -> (-44.6138, 140.4435) centre (-42.5872, 143.7721) ccw projected
  spline S0 degree 2 poles (-44.8154, 140.575) (-46.7745, 145.139) (-50.2264, 149.2557) knots 0 0 0 1 1 1 projected
  arc A7 (-50.2264, 149.2557) -> (-54.8964, 147.6019) centre (0, 0) ccw projected
  arc A8 (-59.2639, 135.1204) -> (-53.6386, 137.4505) centre (-57.3822, 138.5329) ccw projected
  arc A9 (-65.5527, 143.188) -> (-70.0243, 141.0551) centre (0, 0) ccw projected
  arc A10 (-73.0632, 128.1854) -> (-67.7123, 131.0907) centre (-71.5485, 131.776) ccw projected
  arc A11 (-80.1608, 135.5514) -> (-84.385, 132.9629) centre (0, 0) ccw projected
  arc A12 (-86.062, 119.846) -> (-81.044, 123.2948) centre (-84.9309, 123.5752) ccw projected
  arc A13 (-93.8907, 126.4298) -> (-97.8211, 123.4139) centre (0, 0) ccw projected
  arc A14 (-98.1178, 110.1936) -> (-93.4879, 114.1479) centre (-97.3828, 114.0206) ccw projected
  arc A15 (-106.5918, 115.9229) -> (-110.1855, 112.5127) centre (0, 0) ccw projected
  arc A16 (-109.0987, 99.3338) -> (-104.9075, 103.7505) centre (-108.7677, 103.2167) ccw projected
  arc A17 (-118.1252, 104.146) -> (-121.3427, 100.3788) centre (0, 0) ccw projected
  arc A18 (-118.8843, 87.3857) -> (-115.1776, 92.2163) centre (-118.9609, 91.2819) ccw projected
  arc A19 (-128.3643, 91.2281) -> (-131.1704, 87.1452) centre (0, 0) ccw projected
  arc A20 (-127.3673, 74.4802) -> (-124.1859, 79.6718) centre (-127.8508, 78.3471) ccw projected
  arc A21 (-137.197, 77.3106) -> (-139.561, 72.9568) centre (0, 0) ccw projected
  arc A22 (-134.4549, 60.7587) -> (-131.8336, 66.2544) centre (-135.3399, 64.5538) ccw projected
  arc A23 (-144.5266, 62.5461) -> (-146.4225, 57.969) centre (0, 0) ccw projected
  arc A24 (-140.0693, 46.3715) -> (-138.0368, 52.1111) centre (-141.3462, 50.0533) ccw projected
  arc A25 (-150.2727, 47.0963) -> (-151.6798, 42.3461) centre (0, 0) ccw projected
  arc A26 (-144.1492, 31.4762) -> (-142.7278, 37.3968) centre (-145.8039, 35.0044) ccw projected
  line L0 (-143.0357, 16.3365) -> (-7.2895, -24.3315) projected
  arc A27 (-7.2895, -24.3315) -> (25.12, 3.7611) centre (0, 0) ccw projected
  line L1 (25.12, 3.7611) -> (3.8231, 146) projected
  arc A28 (3.4736, 146.0249) -> (3.8231, 146) centre (3.9252, 149.8956) ccw projected
  line L2 (3.6892, 154.4581) -> (25.147, 3.5763)
  arc A29 (-7.2895, -24.3315) -> (25.12, 3.7611) centre (0, 0) ccw projected
  arc A30 (-154.3724, 31.1305) -> (-155.2752, 26.2593) centre (0, 0) ccw projected
  arc A31 (-144.8005, 19.0634) -> (-145.8549, 22.2728) centre (-148.6641, 19.572) ccw projected
  arc A32 (-144.8005, 19.0634) -> (-143.0357, 16.3365) centre (-142.3168, 18.7364) ccw projected
  point P0 (3.4736, 146.0249)
  point P1 (-50.2264, 149.2557)
  point P2 (-44.6138, 140.4435)
  constraints: 5 point on circle, 4 tangent, 2 end point, 1 centre point, 22 other
extrude "Extrusion18" add sketch "Sketch17" against normal blind 6.35 contours A0 L2 L1 A28 | A0 A6 S0 A1
sketch "Sketch20" plane through (6.35, 0, 0) normal (1, 0, 0) x (0, 0, -1)
  circle A0 centre (-21.4577, 150.8818) radius 14.2875 construction
  line L0 (-21.4577, 150.8818) -> (-193.8348, 370.7693) construction
  line L1 (-21.4577, 150.8818) -> (0, 0) construction
  circle A1 centre (-193.8348, 370.7693) radius 14.2875
  circle A2 centre (-193.8348, 370.7693) radius 25.4 construction
  arc A3 (-21.4577, 150.8818) -> (-193.8348, 370.7693) centre (-298.0744, 111.5427) ccw construction
  arc A4 (-46.6047, 147.3055) -> (-203.3111, 347.2033) centre (-298.0744, 111.5427) ccw
  arc A5 (3.6892, 154.4581) -> (-184.3585, 394.3354) centre (-298.0744, 111.5427) ccw
  line L2 (-46.6047, 147.3055) -> (3.6892, 154.4581)
  arc A6 (-184.3585, 394.3354) -> (-203.3111, 347.2033) centre (-193.8348, 370.7693) ccw
  circle A7 centre (-21.4577, 150.8818) radius 14.2875 projected
  circle A8 centre (0, 0) radius 14.2875 projected
  arc A9 (3.6892, 154.4581) -> (-46.7086, 153.6299) centre (-21.4577, 150.8818) ccw projected
  arc A10 (-50.2264, 149.2557) -> (-46.7086, 153.6299) centre (-51.8881, 154.1936) ccw projected
  arc A11 (-50.2264, 149.2557) -> (-54.8964, 147.6019) centre (0, 0) ccw projected
  arc A12 (-59.2639, 135.1204) -> (-53.6386, 137.4505) centre (-57.3822, 138.5329) ccw projected
  arc A13 (-65.5527, 143.188) -> (-70.0243, 141.0551) centre (0, 0) ccw projected
  arc A14 (-73.0632, 128.1854) -> (-67.7123, 131.0907) centre (-71.5485, 131.776) ccw projected
  arc A15 (-80.1608, 135.5514) -> (-84.385, 132.9629) centre (0, 0) ccw projected
  arc A16 (-86.062, 119.846) -> (-81.044, 123.2948) centre (-84.9309, 123.5752) ccw projected
  arc A17 (-93.8907, 126.4298) -> (-97.8211, 123.4139) centre (0, 0) ccw projected
  arc A18 (-98.1178, 110.1936) -> (-93.4879, 114.1479) centre (-97.3828, 114.0206) ccw projected
  arc A19 (-106.5918, 115.9229) -> (-110.1855, 112.5127) centre (0, 0) ccw projected
  arc A20 (-109.0987, 99.3338) -> (-104.9075, 103.7505) centre (-108.7677, 103.2167) ccw projected
  arc A21 (-118.1252, 104.146) -> (-121.3427, 100.3788) centre (0, 0) ccw projected
  arc A22 (-118.8843, 87.3857) -> (-115.1776, 92.2163) centre (-118.9609, 91.2819) ccw projected
  arc A23 (-128.3643, 91.2281) -> (-131.1704, 87.1452) centre (0, 0) ccw projected
  arc A24 (-127.3673, 74.4802) -> (-124.1859, 79.6718) centre (-127.8508, 78.3471) ccw projected
  arc A25 (-137.197, 77.3106) -> (-139.561, 72.9568) centre (0, 0) ccw projected
  arc A26 (-134.4549, 60.7587) -> (-131.8336, 66.2544) centre (-135.3399, 64.5538) ccw projected
  arc A27 (-144.5266, 62.5461) -> (-146.4225, 57.969) centre (0, 0) ccw projected
  arc A28 (-140.0693, 46.3715) -> (-138.0368, 52.1111) centre (-141.3462, 50.0533) ccw projected
  arc A29 (-150.2727, 47.0963) -> (-151.6798, 42.3461) centre (0, 0) ccw projected
  arc A30 (-144.1492, 31.4762) -> (-142.7278, 37.3968) centre (-145.8039, 35.0044) ccw projected
  arc A31 (-154.3724, 31.1305) -> (-155.2752, 26.2593) centre (0, 0) ccw projected
  arc A32 (-144.8005, 19.0634) -> (-145.8549, 22.2728) centre (-148.6641, 19.572) ccw projected
  arc A33 (-144.8005, 19.0634) -> (-143.0357, 16.3365) centre (-142.3168, 18.7364) ccw projected
  line L3 (-143.0357, 16.3365) -> (-7.2895, -24.3315) projected
  arc A34 (-7.2895, -24.3315) -> (25.147, 3.5763) centre (0, 0) ccw projected
  line L4 (25.147, 3.5763) -> (3.6892, 154.4581) projected
  point P0 (-47.2792, 151.7641)
  point P1 (3.6892, 154.4581)
  dimension "d130" = 279.4
  dimension "d131" = 150
  dimension "d132" = 28.575
  dimension "d133" = 50.8
  constraints: 10 point on circle, 6 centre point, 6 end point, 4 tangent, 2 coincident, 1 midpoint, 21 other
  measures "d130" distance of L0.start L0.end
  measures "d131" angle of L1 L0
  measures "d132" diameter of A1
  measures "d133" diameter of A2
extrude "Extrusion21" add sketch "Sketch20" against normal blind 6.35 contours A4 A6 A5 A9 A10
fillet "Fillet1" radius 4.445 1 edges at (3.175, 151.7641, 47.2792)
equation "\"PD\" = 304.8"
equation "\"a\" = 14.5deg"
equation "\"add\" = mod"
equation "\"ded\" = 6.35"
equation "\"RD\" = PD - 2 * ded"
equation "\"OD\" = PD + 2 * add"
equation "\"mod\" = 5.08"
body "Solid2"
